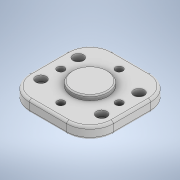
# Autodesk Inventor part: schunk_egi_quick_release_adapter_plate
Saved by Autodesk Inventor 2020 (Build 240168000, 168)
## iProperties
Created: 2021-03-02
Part Number: schunk_egi_quick_release_adapter_plate
Material: Generic
Document SubType Name: Modeling
Designer: NILY
Density: 1 g/cm^3
Appearance: Default
Author: NILY
Autodesk Inventor part; units mm, degrees
ref_plane "YZ Plane" through (0, 0, 0) normal (1, 0, 0) x (0, 1, 0)
ref_plane "XZ Plane" through (0, 0, 0) normal (0, 1, 0) x (-1, 0, 0)
ref_plane "XY Plane" through (0, 0, 0) normal (0, 0, 1) x (1, 0, 0)
sketch "Sketch1" plane through (0, 0, 0) normal (0, 1, 0) x (-1, 0, 0)
  line L0 (36, -36) -> (-36, -36)
  line L1 (-36, -36) -> (-36, 36)
  line L2 (-36, 36) -> (36, 36)
  line L3 (36, 36) -> (36, -36)
  point P0 (36, 0)
  point P1 (0, 0)
  point P2 (0, -36)
  dimension "d4" = 72
  dimension "d5" = 72
  constraints: 8 end point, 2 midpoint, 2 parallel, 1 horizontal, 1 horizontal alignment, 1 perpendicular, 1 vertical alignment
  measures "d4" distance of L1.end L2.end
  measures "d5" distance of L0.end L1.end
extrude "Extrusion1" add sketch "Sketch1" along normal blind 10
sketch "Sketch2" plane through (0, 10, 0) normal (0, 1, 0) x (1, 0, 0)
  point P0 (0, 0)
  point P1 (-26, -16)
  dimension "d13" = 16
  dimension "d14" = 26
  measures "d13" vertical distance of point (0, 0) point (-26, -16)
  measures "d14" horizontal distance of point (0, 0) point (-26, -16)
hole "Hole1" at (-26, 10, 16) direction (0, -1, 0) diameter 5.5 end through all counterbore diameter 9 counterbore depth 5 clearance for "Hex Head Bolt" size "M5" standard "Ansi Metric M Profile"
pattern_linear "Rectangular Pattern1" count 2 spacing 52 along (1, 0, 0) count 2 spacing 32 along (0, 0, -1) of "Hole1"
sketch "Sketch3" plane through (0, 10, 0) normal (0, 1, 0) x (1, 0, 0)
  point P0 (0, 0)
  point P1 (0, 25)
  dimension "d28" = 25
  constraints: 1 vertical alignment
  measures "d28" distance of point (0, 0) point (0, 25)
hole "Hole2" at (0, 10, -25) direction (0, -1, 0) diameter 6.3 end through all clearance for "Hex Head Bolt" size "M6" standard "Ansi Metric M Profile"
sketch "Sketch5" plane through (0, 0, 0) normal (0, -1, 0) x (1, 0, 0)
  circle A0 centre (0, -25) radius 3.15 projected
  line L0 (-2.8911, -20.0025) -> (2.8824, -19.9975)
  line L1 (2.8824, -19.9975) -> (5.7735, -24.995)
  line L2 (5.7735, -24.995) -> (2.8911, -29.9975)
  line L3 (2.8911, -29.9975) -> (-2.8824, -30.0025)
  line L4 (-2.8824, -30.0025) -> (-5.7735, -25.005)
  line L5 (-5.7735, -25.005) -> (-2.8911, -20.0025)
  point P0 (0, 0)
  dimension "d38" = 10
  constraints: 12 end point, 1 coincident, 13 other
  measures "d38" distance between parallel lines of L5 L2
extrude "Extrusion3" cut sketch "Sketch5" against normal blind 5 contours A0 | L0 L1 L2 L3 L4 L5
pattern_circular "Circular Pattern3" count 4 over 360 about axis through (0, -10, 0) along (0, 1, 0) of "Hole2", "Extrusion3"
sketch "Sketch6" plane through (0, 10, 0) normal (0, 1, 0) x (1, 0, 0)
  circle A0 centre (0, 0) radius 15.5
  dimension "d44" = 31
  constraints: 1 centre point, 1 coincident
  measures "d44" diameter of A0
extrude "Extrusion4" add sketch "Sketch6" along normal blind 4
chamfer "Chamfer1" distance 1 angle 45 1 edges at (-15.5, 14, 0)
fillet "Fillet1" radius 20 4 edges at (-36, 5, 36) (36, 5, 36) (36, 5, -36) (-36, 5, -36)
fillet "Fillet2" radius 2 16 edges at (30.1421, 10, 30.1421) (36, 10, 0) (30.1421, 10, -30.1421) (0, 10, -36) (-30.1421, 10, -30.1421) (-36, 10, 0) (-30.1421, 10, 30.1421) (0, 10, 36) (30.1421, 0, 30.1421) (36, 0, 0) (30.1421, 0, -30.1421) (0, 0, -36) (-30.1421, 0, -30.1421) (-36, 0, 0) (-30.1421, 0, 30.1421) (0, 0, 36)
body "Solid1"
